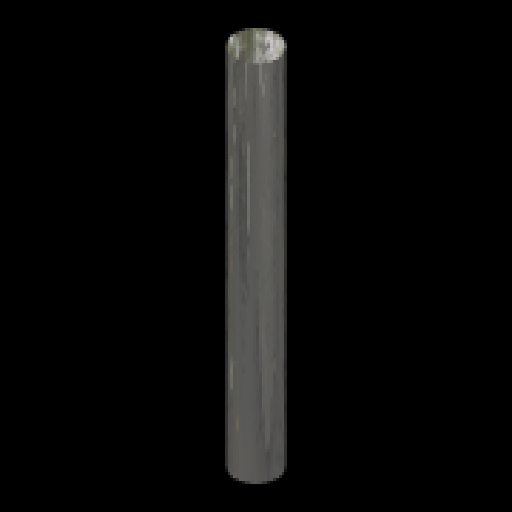
# Autodesk Inventor part: ShaftPlaceholder
Saved by Autodesk Inventor 2023 (Build 270158030, 158C)
## iProperties
Created: 2022-11-17
Part Number: ShaftPlaceholder
Material: Steel, Alloy
Document SubType Name: Modeling
Designer: kumpu
Density: 7.73 g/cm^3
Appearance: Semi-Polished
Author: kumpu
Autodesk Inventor part; units mm, degrees
ref_plane "YZ Plane" through (0, 0, 0) normal (1, 0, 0) x (0, 1, 0)
ref_plane "XZ Plane" through (0, 0, 0) normal (0, 1, 0) x (-1, 0, 0)
ref_plane "XY Plane" through (0, 0, 0) normal (0, 0, 1) x (1, 0, 0)
sketch "Sketch1" plane through (0, 0, 0) normal (0, 1, 0) x (-1, 0, 0)
  circle A0 centre (0, 0) radius 12.7
  dimension "d0" = 25.4
  constraints: 1 centre point, 1 coincident
  measures "d0" diameter of A0
extrude "Extrusion1" add sketch "Sketch1" along normal blind 215.9
body "Solid1"
